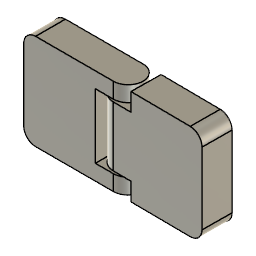
Hinge_f3d (Autodesk Fusion 360 design; units mm, degrees)
part number: 2025-10-24-17-26-06-746
part number: 2025-10-24-18-00-21-172
part number: 2025-10-24-18-07-09-223
Autodesk Fusion 360 part; units mm, degrees
sketch "Sketch1" plane through (0, 0, 0) normal (0, 0, 1) x (1, 0, 0)
  line L0 (-15, 0) -> (0, 0)
  line L1 (0, 5) -> (-15, 5)
  line L2 (-15, 5) -> (-15, 0)
  arc A0 (0, 0) -> (0, 5) centre (0, 2.5) ccw
  circle A1 centre (0, 2.5) radius 1.35
  circle A2 centre (0, 2.5) radius 1.75
  line L3 (-3, 5) -> (-3, 0)
  dimension "d3" = 15
  dimension "d4" = 5
  dimension "d6" = 3.5
  dimension "d8" = 2.7
  dimension "d10" = 12
  constraint horizontal L0
  constraint horizontal L1
  constraint vertical L2
  constraint coincident L0 A0.start
  constraint tangent L0 A0
  constraint tangent L1 A0
  constraint concentric A0 A1
  constraint concentric A1 A2
  constraint coincident L1 L3.start
  constraint coincident L0 L3.end
  constraint perpendicular L0 L3
  measures "d3" distance of L1.start L1.end
  measures "d4" distance of L0.start L1.end
  measures "d6" diameter of A2
  measures "d8" diameter of A1
  measures "d10" distance of L2 L3
extrude "Extrude1" add sketch "Sketch1" along normal blind 2.6 contours L0 L1 L2 L3 | L0 L1 A0 L3 | A1 | A2 makes body 1
extrude "Extrude2" add sketch "Sketch1" along normal blind 8 contours L0 L1 L2 L3 | A1 bodies 1
ref_plane "WorkPlane1" through (0, 2.5, 8) normal (0, 0, 1) x (1, 0, 0)
mirror "Mirror1" about plane through (0, 2.5, 8) normal (0, 0, 1) of bodies 1 merged
copy_body "Body->Comp1" bodies 1 removing the originals makes body 2 in component "Component"
extrude "Extrude3" add sketch "Sketch1" along normal blind 10 separate body contours L0 L1 L2 L3 | L0 L1 A0 L3 makes body 3
extrude "Extrude4" add sketch "Sketch1" against normal blind 3 separate body contours L0 L1 L2 L3 makes body 4
ref_plane "WorkPlane2" through (-6.25, 2.5, 5) normal (0, 0, 1) x (1, 0, 0)
mirror "Mirror2" about plane through (-6.25, 2.5, 5) normal (0, 0, 1) of bodies 4 makes body 5
combine "Combine1" operation add target body 5 tool bodies 4 3
copy_body "Body->Comp2" bodies 5 removing the originals makes body 6 in component "Component'"
move_body "Move1" bodies 2 to x (1, 0, 0) y (0, 1, 0) z (0, 0, 1) at (20, 0, 0) in component "Component"
fillet "Fillet1" radius 2 2 edges at (5, 2.5, 0) (5, 2.5, 16) on bodies 2 in component "Component"
fillet "Fillet1'" radius 2 2 edges at (-15, 2.5, 13) (-15, 2.5, -3) on bodies 6 in component "Component'"
component "Component" placed x (1, 0, 0) y (0, 1, 0) z (0, 0, 1) at (0, 0, 0)
component "Component'" placed x (1, 0, 0) y (0, 1, 0) z (0, 0, 1) at (20, 0, 3)
equation "d_length = 15 mm"
equation "d_width = 5 mm"
equation "d3 = d_length"
equation "d4 = d_width"
equation "outer_circle_dia = 3.5 mm"
equation "d6 = outer_circle_dia"
equation "tol = 0.4 mm"
equation "d8 = outer_circle_dia - 2 * tol"
equation "d_inner_len = 12 mm"
equation "d10 = d_inner_len"
equation "curl_thick = 3 mm"
equation "d12 = curl_thick - tol"
equation "shaft_length = 10 mm"
equation "d15 = curl_thick + shaft_length / 2"
equation "d20 = shaft_length"
equation "d22 = -curl_thick"
